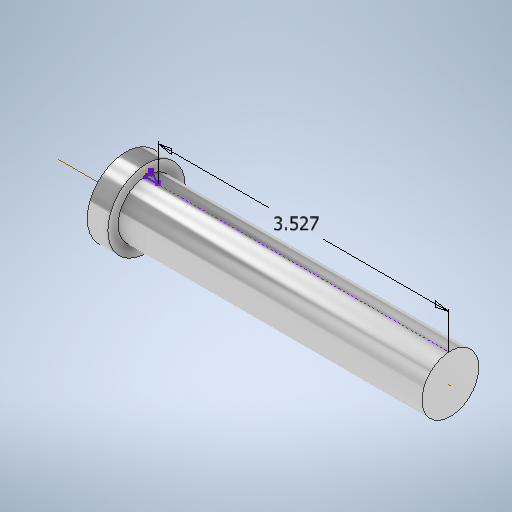
# Autodesk Inventor part: Part2
Saved by Autodesk Inventor 2025.1 (Build 291241000, 241)
## iProperties
Created: 2024-08-17
Part Number: Part2
Material: Generic
Document SubType Name: Modeling
Designer: vedan
Density: 1 g/cm^3
Appearance: Chrome - Polished
Author: vedan
Autodesk Inventor part; units mm, degrees
ref_plane "YZ Plane" through (0, 0, 0) normal (1, 0, 0) x (0, 1, 0)
ref_plane "XZ Plane" through (0, 0, 0) normal (0, 1, 0) x (-1, 0, 0)
sketch "Sketch1" plane through (0, 0, 0) normal (0, 1, 0) x (-1, 0, 0)
  line L0 (64.106, 4.246) -> (64.106, -7.6666)
  line L1 (-35.9192, -4.517) -> (-35.9192, 4.246)
  line L2 (-35.9192, 4.246) -> (64.106, 4.246)
  line L3 (24.879, -4.517) -> (-35.9192, -4.517)
  line L4 (-35.9192, -4.517) -> (-35.9192, 4.246)
  line L5 (-35.9192, 4.246) -> (64.106, 4.246)
  line L6 (57.756, -7.6666) -> (64.106, -7.6666)
  line L7 (64.106, -7.6666) -> (57.756, -7.6666)
  line L8 (57.756, -7.6666) -> (57.756, -4.517)
  line L9 (57.756, -4.517) -> (24.879, -4.517)
  point P0 (0, 0)
  dimension "d4" = 11.9126
  dimension "d5" = 100.0252
  dimension "d6" = 6.35
  dimension "d7" = 3.1496
  constraints: 20 end point, 2 collinear, 2 perpendicular, 1 horizontal, 1 parallel, 1 vertical
  measures "d4" distance of L0.start L0.end
  measures "d5" distance of L1.end L0.start
  measures "d6" distance of L6.start L0.end
  measures "d7" distance of L6.start L8.end
revolve "Revolution1" add sketch "Sketch1" angle 360 about axis through (35.9192, 0, 4.246) along (-1, 0, 0)
ref_plane "Work Plane3" through (0, 0, 4.7625) normal (0, 0, 1) x (1, 0, 0)
sketch "Sketch8" plane through (0, 0, 4.7625) normal (0, 0, 1) x (1, 0, 0)
  line L0 (-55.7252, 11.3974) -> (-55.7252, 7.4576) construction
  line L1 (-53.6658, 8.763) -> (35.9192, 8.763) construction
  line L2 (35.9192, 8.763) -> (-57.756, 8.763) construction
  line L3 (-56.0328, 10.9296) -> (-57.5509, 8.8518)
  arc A0 (-57.756, 8.7476) -> (-57.5509, 8.8518) centre (-57.756, 9.0016) ccw
  line L4 (-55.4175, 10.9296) -> (-53.8995, 8.8518)
  arc A1 (-53.8995, 8.8518) -> (-53.6944, 8.7476) centre (-53.6944, 9.0016) ccw
  arc A2 (-55.4175, 10.9296) -> (-56.0328, 10.9296) centre (-55.7252, 10.7048) ccw
  line L5 (-56.7919, 9.9061) -> (-54.6585, 9.9061) construction
  line L6 (-57.756, 11.9126) -> (-57.756, -11.9126) construction
  line L7 (-57.756, 8.7476) -> (-51.4573, 8.7476) construction
  line L8 (-53.6944, 8.7476) -> (-57.756, 8.7476)
  point P0 (0, 0)
  point P1 (-40.5643, 2.2991)
  point P2 (-41.4145, 2.2991)
  point P3 (-55.7252, 11.366)
  point P4 (-57.6499, 8.763)
  dimension "d53" = 89.585
  constraints: 14 end point, 6 point on circle, 4 point on line, 4 tangent, 3 centre point, 1 collinear, 1 parallel, 1 vertical
  measures "d53" distance of L1.end L1.start
body "Solid1"
